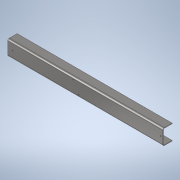
# Autodesk Inventor part: SlipersLåda 211018001
Saved by Autodesk Inventor 2020 (Build 240168000, 168)
## iProperties
Created: 2021-10-18
Part Number: SlipersLåda 211018001
Material: Steel, Mild
Document SubType Name: Sheet Metal
Designer: dicpet001
Density: 7.85 g/cm^3
Sheet Metal Rule: Default_mm
Appearance: Semi-Polished
Author: dicpet001
Autodesk Inventor part; units mm, degrees
ref_plane "YZ Plane" through (0, 0, 0) normal (1, 0, 0) x (0, 1, 0)
ref_plane "XZ Plane" through (0, 0, 0) normal (0, 1, 0) x (-1, 0, 0)
ref_plane "XY Plane" through (0, 0, 0) normal (0, 0, 1) x (1, 0, 0)
sketch "Sketch1" plane through (0, 0, 0) normal (0, 0, 1) x (1, 0, 0)
  line L0 (0, 196) -> (0, -196)
  line L1 (-2100, 0) -> (2100, 0)
  line L2 (-1500, 140) -> (1500, 140)
  line L3 (1500, 140) -> (1500, -140)
  line L4 (1500, -140) -> (-1500, -140)
  line L5 (-1500, -140) -> (-1500, 140)
  point P0 (0, 0)
  dimension "d0" = 3000
  dimension "d1" = 280
  measures "d0" distance of L2.start L2.end
  measures "d1" distance of L2.end L3.end
extrude "Plate1" add sketch "Sketch1" against normal blind 10
sketch "Sketch2" plane through (1500, 140, -10) normal (0, 1, 0) x (-1, 0, 0)
  line L0 (3000, 0) -> (0, 0)
  line L1 (0, 0) -> (0, -170)
  line L2 (0, -170) -> (3000, -170)
  line L3 (3000, -170) -> (3000, 0)
  constraints: 6 end point, 1 horizontal, 1 perpendicular, 1 vertical
edge flange "Flange1" height 180 angle 90 thickness 10 bend radius 20 thickness toward (0, 1, 0) relief straight relief width 10 relief depth 5 corner gap 10 corner form 0 edges at (0, 140, -10) (0, -140, -10) wall of the first edge with corners at (-1500, 140, -10) (1500, 140, -10) (1500, 140, -180) (-1500, 140, -180)
bend "Bend1"
corner "Corner1"
chamfer "Chamfer1" [suppressed]
sketch "Sketch3" plane through (0, 0, -10) normal (0, 0, -1) x (-1, 0, 0)
  line L0 (1500, 120) -> (1500, -120) projected
  line L1 (-1500, -120) -> (-1500, 120) projected
  line L2 (-1500, 150) -> (1500, 150) projected
  line L3 (1500, -150) -> (-1500, -150) projected
  line L4 (303.3431, 108.3365) -> (61.6569, 108.3365) projected
  line L5 (-1500, -120) -> (1500, -120) projected
  line L6 (1500, 120) -> (-1500, 120) projected
  point P0 (0, 0)
  point P1 (1405, 0)
  point P2 (-1455, 0)
  point P3 (235, 100)
  point P4 (130, -100)
  dimension "d16" = 45
  dimension "d17" = 95
  dimension "d18" = 105
  dimension "d19" = 130
  dimension "d20" = 100
  dimension "d29" = 100
  measures "d16" distance from line of L1 point (-1455, 0)
  measures "d17" distance from line of point (1405, 0) L0
  measures "d18" horizontal distance of point (130, -100) point (235, 100)
  measures "d19" horizontal distance of point (130, -100) point (0, 0)
  measures "d20" vertical distance of point (0, 0) point (130, -100)
  measures "d29" vertical distance of point (235, 100) point (0, 0)
hole "Hole1" at (-1405, 0, -10) at (1455, 0, -10) at (-235, 100, -10) at (-130, -100, -10) direction (0, 0, 1) diameter 18.631 end through all thread size "G20.955x1.814" designation "G 1/2" standard "GB Pipe Threads without seal"
sketch "Sketch4" plane through (-1500, 140, 170) normal (0, -1, 0) x (1, 0, 0)
  line L0 (3000, -150) -> (0, -150) projected
  line L1 (3000, -180) -> (3000, -150) projected
  line L2 (0, -180) -> (3000, -180) projected
  line L3 (0, -150) -> (0, -180) projected
  line L4 (3000, -9) -> (0, -9) projected
  line L5 (3000, -150) -> (3000, -9) projected
  line L6 (3000, -150) -> (0, -150) projected
  line L7 (0, -9) -> (0, -150) projected
  point P0 (1500, -170)
  point P1 (2950, -64)
  point P2 (2649, -120)
  dimension "d30" = 50
  dimension "d31" = 116
  dimension "d32" = 351
  dimension "d33" = 60
  measures "d30" distance from line of point (2950, -64) L5
  measures "d31" distance from line of point (2950, -64) L2
  measures "d32" distance from line of L5 point (2649, -120)
  measures "d33" distance from line of L2 point (2649, -120)
hole "Hole2" [suppressed]
equation "\"d2\" = Thickness"
equation "\"d3\" = BendReliefWidth"
equation "\"d4\" = BendReliefDepth"
equation "\"d5\" = MinimumRemnant"
equation "\"d6\" = TransitionRadius"
equation "\"d10\" = CornerReliefSize"
equation "\"d11\" = GapSize"
equation "\"d12\" = JacobiRadiusSize"
equation "\"BendReliefDepth\" = 0.5 * Thickness"
equation "\"Thickness\" = 10"
equation "\"BendReliefWidth\" = 10"
equation "\"MinimumRemnant\" = 20"
equation "\"TransitionRadius\" = 10"
equation "\"CornerReliefSize\" = 40"
equation "\"GapSize\" = 10"
equation "\"JacobiRadiusSize\" = 10"
body "Solid1"
